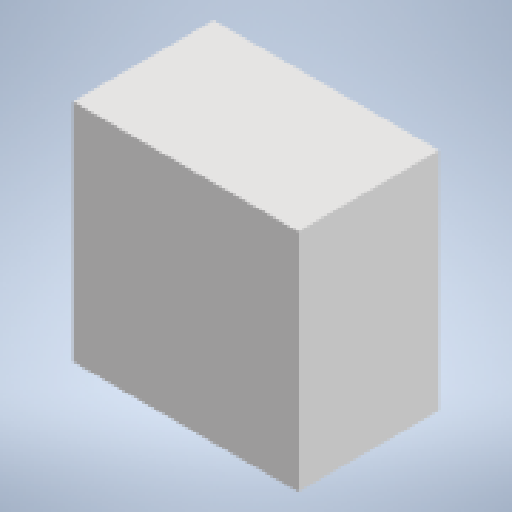
# Autodesk Inventor part: Caja
Saved by Autodesk Inventor 2023 (Build 270158000, 158)
## iProperties
Created: 2023-04-03
Part Number: Caja
Material: Genérico
Document SubType Name: Modeling
Designer: sergi
Density: 1 g/cm^3
Appearance: Valor por defecto
Author: sergi
Autodesk Inventor part; units mm, degrees
ref_plane "YZ Plane" through (0, 0, 0) normal (1, 0, 0) x (0, 1, 0)
ref_plane "XZ Plane" through (0, 0, 0) normal (0, 1, 0) x (-1, 0, 0)
ref_plane "XY Plane" through (0, 0, 0) normal (0, 0, 1) x (1, 0, 0)
sketch "Boceto1" plane through (0, 0, 0) normal (0, 0, 1) x (1, 0, 0)
  circle A0 centre (-35.8, -35.8) radius 2.125 projected
  circle A1 centre (35.8, 35.8) radius 2.125 projected
  circle A2 centre (35.8, -35.8) radius 2.125 projected
  circle A3 centre (-35.8, 35.8) radius 2.125 projected
  line L0 (-40, -40) -> (-40, 40) projected
  line L1 (40, -40) -> (-40, -40) projected
  line L2 (40, 40) -> (40, -40) projected
  line L3 (-40, 40) -> (40, 40) projected
  line L4 (-40, 40) -> (40, 40)
  line L5 (40, 40) -> (40, -40)
  line L6 (40, -40) -> (-40, -40)
  line L7 (-40, -40) -> (-40, 40)
  line L8 (-41, -41) -> (-41, 41)
  line L9 (-41, 41) -> (41, 41)
  line L10 (41, 41) -> (41, -41)
  line L11 (41, -41) -> (-41, -41)
  point P0 (0, 0)
  dimension "d22" = 1
  constraints: 16 end point, 2 parallel, 1 horizontal, 1 perpendicular, 3 other
  measures "d22" distance between parallel lines of L1 L11
extrude "Extrusión1" add sketch "Boceto1" along normal blind 50 contours A0 | A1 | A2 | A3 | L0 L3 L2 L1
sketch "Boceto2" plane through (0, 0, 0) normal (0, 0, -1) x (-1, 0, 0)
  circle A0 centre (35.8, 35.8) radius 2.125 projected
  circle A1 centre (35.8, -35.8) radius 2.125 projected
  circle A2 centre (-35.8, -35.8) radius 2.125 projected
  circle A3 centre (-35.8, 35.8) radius 2.125 projected
  point P0 (0, 0)
hole "Agujero1" at (-35.8, 35.8, 0) at (-35.8, -35.8, 0) at (35.8, -35.8, 0) at (35.8, 35.8, 0) direction (0, 0, 1) diameter 4.25 depth 10
shell "Vaciado1" thickness 1.6 removed faces 2 at (11.4636, -11.4031, 0) at (13.3333, 40, 16.6667)
sketch "Boceto3" plane through (37.8, 37.8, 48.4) normal (0, 0, -1) x (-1, 0, 0)
  circle A0 centre (65.77, -19.059) radius 1.4999 projected
  circle A1 centre (62.025, -68.7162) radius 1.5 projected
  line L0 (76.2, 2.2) -> (76.2, -76.2) projected
  line L1 (-0.6, -76.2) -> (-0.6, 2.2) projected
  line L2 (76.2, -76.2) -> (-0.6, -76.2) projected
  circle A2 centre (7.8236, -54.3604) radius 1.5 projected
  circle A3 centre (7.2748, -21.6806) radius 1.5001 projected
  circle A4 centre (65.77, -19.059) radius 3
  circle A5 centre (62.025, -68.7162) radius 3
  circle A6 centre (7.8236, -54.3604) radius 3
  circle A7 centre (7.2748, -21.6806) radius 3
  line L3 (-0.6, 2.2) -> (76.2, 2.2) projected
  point P0 (37.8, -37.8)
  dimension "d10" = 6
  dimension "d11" = 6
  dimension "d12" = 6
  dimension "d13" = 6
  constraints: 4 centre point, 4 coincident
  measures "d10" diameter of A4
  measures "d11" diameter of A5
  measures "d12" diameter of A6
  measures "d13" diameter of A7
extrude "Extrusión2" add sketch "Boceto3" along normal blind 5 contours A4 | A5 | A6 | A7
fillet "Empalme1" radius 2 4 edges at (-21.225, -30.9162, 48.4) (32.9764, -16.5604, 48.4) (33.5252, 16.1194, 48.4) (-24.97, 18.741, 48.4)
sketch "Boceto4" plane through (-38.4, -38.4, 48.4) normal (1, 0, 0) x (0, 0, -1)
  line L0 (14.2955, 15.5019) -> (14.2955, 22.9876) projected
  line L1 (14.2955, 22.9876) -> (7, 23.1181) projected
  line L2 (7, 15.5019) -> (14.2955, 15.5019) projected
  line L3 (14.2955, 15.5019) -> (7, 15.5019)
  line L4 (7, 15.5019) -> (7, 23.1181)
  line L5 (7, 23.1181) -> (14.2955, 23.1181)
  line L6 (14.2955, 23.1181) -> (14.2955, 15.5019)
  line L7 (6, 24.1181) -> (6, 14.5019)
  line L8 (6, 14.5019) -> (15.2955, 14.5019)
  line L9 (15.2955, 14.5019) -> (15.2955, 24.1181)
  line L10 (15.2955, 24.1181) -> (6, 24.1181)
  point P0 (48.4, 38.4)
  point P1 (14.2955, 22.9876)
  point P2 (10.9796, 28.9019)
  dimension "d17" = 1
  constraints: 16 end point, 4 parallel, 2 perpendicular, 1 horizontal, 3 other
  measures "d17" distance between parallel lines of L4 L7
extrude "Extrusión3" cut sketch "Boceto4" against normal blind 5 contours L2 L4 L1 L0 | L1 L5 L6 | L10 L9 L8 L7
sketch "Boceto5" plane through (-40, 40, 0) normal (0, 1, 0) x (1, 0, 0)
  line L0 (0, -50) -> (80, -50) projected
  line L1 (0, -50) -> (80, -50)
  line L2 (80, -50) -> (80, 25.124)
  line L3 (80, 25.124) -> (0, 25.124)
  line L4 (0, 25.124) -> (0, -50)
  point P0 (40, 0)
  constraints: 8 end point, 2 parallel, 1 horizontal, 1 perpendicular
extrude "Extrusión4" add sketch "Boceto5" along normal blind 2
sketch "Boceto6" plane through (-40, 42, 0) normal (0, 1, 0) x (1, 0, 0)
  line L0 (80, 25.124) -> (0, 25.124) projected
  line L1 (80, -50) -> (80, 25.124) projected
  line L2 (0, 25.124) -> (80, 25.124)
  line L3 (80, 25.124) -> (80, 22.124)
  line L4 (80, 22.124) -> (0, 22.124)
  line L5 (0, 22.124) -> (0, 25.124)
  point P0 (40, 0)
  dimension "d25" = 3
  constraints: 8 end point, 2 parallel, 1 horizontal, 1 perpendicular, 1 point on line
  measures "d25" distance of L2.end L3.end
extrude "Extrusión5" add sketch "Boceto6" along normal blind 15
sketch "Boceto7" plane through (40, 40, -25.124) normal (0, 0, -1) x (-1, 0, 0)
  line L0 (0, 2) -> (80, 2) projected
  line L1 (80, 0) -> (80, 17) projected
  point P0 (40, -40)
  point P1 (70, 11.3)
  dimension "d28" = 9.3
  dimension "d29" = 10
  measures "d28" distance from line of L0 point (70, 11.3)
  measures "d29" distance from line of L1 point (70, 11.3)
hole "Agujero2" at (-30, 51.3, -25.124) direction (0, 0, 1) diameter 5 depth 10
sketch "Boceto8" plane through (40, 40, -25.124) normal (0, 0, -1) x (-1, 0, 0)
  line L0 (0, 2) -> (80, 2) projected
  line L1 (0, 0) -> (0, 17) projected
  point P0 (40, -40)
  point P1 (10, 11.3)
  dimension "d37" = 9.3
  dimension "d38" = 10
  measures "d37" distance from line of L0 point (10, 11.3)
  measures "d38" distance from line of L1 point (10, 11.3)
hole "Agujero3" at (30, 51.3, -25.124) direction (0, 0, 1) diameter 5 depth 10
fillet "Empalme2" radius 3 6 edges at (-40, 42, 13.938) (-40, -40, 25) (40, 42, 13.938) (40, -40, 25) (-40, 57, -23.624) (40, 57, -23.624)
sketch "Boceto9" plane through (-38.4, -33.1325, 0) normal (1, 0, 0) x (0, 0, -1)
  line L0 (-32.0511, 38.9222) -> (-32.0511, 48.6464) projected
  line L1 (-32.0511, 48.6464) -> (-43.4, 48.6464) projected
  line L2 (-32.0511, 48.6464) -> (-32.0511, 73.1325)
  line L3 (-48.4, 73.1325) -> (0, 73.1325) projected
  line L4 (-32.0511, 48.6464) -> (-7.565, 48.6464) construction
  line L5 (-32.0511, 73.1325) -> (-32.0511, 71.1325)
  line L6 (-32.0511, 71.1325) -> (-32.0511, 61.6325)
  line L7 (-32.0511, 61.6325) -> (-43.5511, 61.6325)
  line L8 (-43.5511, 61.6325) -> (-43.5511, 71.1325)
  line L9 (-43.5511, 71.1325) -> (-32.0511, 71.1325)
  line L10 (-32.0511, 71.1325) -> (-32.0511, 61.6325)
  point P0 (0, 33.1325)
  dimension "d47" = 90
  dimension "d48" = 2
  dimension "d49" = 9.5
  dimension "d50" = 11.5
  constraints: 16 end point, 3 point on line, 2 horizontal, 2 parallel, 2 perpendicular
  measures "d47" angle of L4 L2
  measures "d48" distance of L2.end L5.end
  measures "d49" distance of L5.end L6.end
  measures "d50" distance of L8.end L9.end
extrude "Extrusión6" cut sketch "Boceto9" against normal blind 15
fillet "Empalme4" radius 2 6 edges at (33.1325, -38.4, 5.8) (38.4, -33.1325, 5.8) (38.4, 33.1325, 5.8) (-38.4, 33.1325, 5.8) (-33.1325, -38.4, 5.8) (-38.4, -33.1325, 5.8)
sketch "Boceto11" plane through (-38.4, -38.4, 48.4) normal (0, 1, 0) x (1, 0, 0)
  line L0 (17.175, 5) -> (11.175, 5) projected
  line L1 (17.175, 5) -> (67.175, 5)
  line L2 (67.175, 5) -> (67.175, 12)
  line L3 (67.175, 12) -> (17.175, 12)
  line L4 (17.175, 12) -> (17.175, 5)
  line L5 (71.3764, 5) -> (65.3764, 5) projected
  point P0 (38.4, 48.4)
  dimension "d58" = 50
  dimension "d59" = 7
  constraints: 8 end point, 2 parallel, 1 horizontal, 1 perpendicular
  measures "d58" distance of L3.end L2.end
  measures "d59" distance of L2.end L1.end
extrude "Extrusión8" cut sketch "Boceto11" against normal blind 4.5
